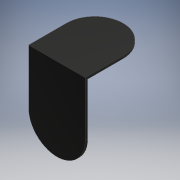
# Autodesk Inventor part: linkage connector
Saved by Autodesk Inventor 2017 (Build 210142000, 142)
## iProperties
Created: 2018-10-18
Part Number: linkage connector
Material: Generic
Document SubType Name: Modeling
Designer: Cameron
Density: 1 g/cm^3
Appearance: Glossy - Black
Author: Cameron
Autodesk Inventor part; units mm, degrees
ref_plane "YZ Plane" through (0, 0, 0) normal (1, 0, 0) x (0, 1, 0)
ref_plane "XZ Plane" through (0, 0, 0) normal (0, 1, 0) x (-1, 0, 0)
ref_plane "XY Plane" through (0, 0, 0) normal (0, 0, 1) x (1, 0, 0)
sketch "Sketch1" plane through (0, 0, 0) normal (0, 1, 0) x (-1, 0, 0)
  line L0 (0, 0) -> (24, 0)
  line L1 (24, 0) -> (24, -35)
  line L2 (0, -35) -> (0, 0)
  arc A0 (0, -23) -> (24, -23) centre (12, -23) ccw
  dimension "d0" = 24
  dimension "d1" = 35
  constraints: 6 end point, 2 point on circle, 2 point on line, 2 tangent, 1 centre point, 1 horizontal, 1 parallel, 1 perpendicular
  measures "d0" distance of L1.end L2.start
  measures "d1" distance of L0.end L1.end
extrude "Extrusion1" add sketch "Sketch1" along normal blind 1
sketch "Sketch2" plane through (0, 1, 0) normal (0, 1, 0) x (1, 0, 0)
  line L0 (-24, 0) -> (0, 0) projected
  line L1 (0, 0) -> (0, 23) projected
  line L2 (-24, 0) -> (0, 0)
  line L3 (0, 0) -> (0, 1)
  line L4 (0, 1) -> (-24, 1)
  line L5 (-24, 1) -> (-24, 0)
  dimension "d4" = 1
  constraints: 8 end point, 2 parallel, 1 horizontal, 1 perpendicular, 1 point on line
  measures "d4" distance of L3.end L2.end
extrude "Extrusion2" add sketch "Sketch2" along normal blind 27
fillet "Fillet1" radius 12 2 edges at (0, 28, -0.5) (-24, 28, -0.5)
body "Solid1"
